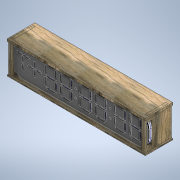
# Autodesk Inventor part: 7 Segment Clock Master
Saved by Autodesk Inventor 2021 (Build 250183000, 183)
## iProperties
Created: 2020-06-26
Part Number: 7 Segment Clock Master
Material: PMMA PlasticBlack
Document SubType Name: Modeling
Designer: dech3
Density: 1.188 g/cm^3
Appearance: Polycarbonate - Clear(1)
Author: dech3
Autodesk Inventor part; units mm, degrees
(part 1 of 5)
ref_plane "YZ Plane" through (0, 0, 0) normal (1, 0, 0) x (0, 1, 0)
ref_plane "XZ Plane" through (0, 0, 0) normal (0, 1, 0) x (-1, 0, 0)
ref_plane "XY Plane" through (0, 0, 0) normal (0, 0, 1) x (1, 0, 0)
sketch "Single Segment" plane through (0, 0, 0) normal (0, 0, 1) x (1, 0, 0)
  arc A0 (128.9839, -2.0293) -> (129.691, -2.3222) centre (129.691, -1.3222) ccw
  arc A1 (129.691, 2.6778) -> (128.9839, 2.3849) centre (129.691, 1.6778) ccw
  line L0 (128.9839, -2.0293) -> (127.0768, -0.1222)
  line L1 (128.9839, 2.3849) -> (127.0768, 0.4778)
  line L2 (127.0768, 0.1778) -> (127.0768, -0.1222)
  line L3 (127.0768, 0.1778) -> (127.0768, 0.4778)
  line L4 (129.691, 2.6778) -> (146.4626, 2.6778)
  line L5 (146.4626, -2.3222) -> (129.691, -2.3222)
  arc A2 (147.1697, 2.3849) -> (146.4626, 2.6778) centre (146.4626, 1.6778) ccw
  line L6 (147.1697, 2.3849) -> (149.0768, 0.4778)
  line L7 (149.0768, 0.1778) -> (149.0768, 0.4778)
  line L8 (149.0768, 0.1778) -> (149.0768, -0.1222)
  arc A3 (146.4626, -2.3222) -> (147.1697, -2.0293) centre (146.4626, -1.3222) ccw
  line L9 (147.1697, -2.0293) -> (149.0768, -0.1222)
  point P0 (153.0768, 0)
  point P1 (129.2768, -2.3222)
  point P2 (129.2768, 2.6778)
  point P3 (146.8768, 2.6778)
  point P4 (146.8768, -2.3222)
  dimension "d105" = 2.2
  dimension "d108" = 2.2
  dimension "d111" = 2.2
  dimension "d112" = 2.2
  dimension "d113" = 2.2
  dimension "d114" = 2.2
  dimension "d115" = 2.2
  dimension "d116" = 1
  dimension "d117" = 5
  dimension "d121" = 2.2
  dimension "d122" = 2.2
  dimension "d126" = 135
  dimension "d127" = 22
  dimension "d128" = 135
  dimension "d129" = 2.5
  dimension "d348" = 5
  dimension "d349" = 22
  dimension "d350" = 2.2
  dimension "d352" = 0.3
  dimension "d353" = 0.3
  dimension "d358" = 0.3
  dimension "d359" = 0.3
  measures "d105" horizontal distance of point (129.277, -2.322) L0.end
  measures "d108" horizontal distance of L7.end point (146.877, 2.678)
  measures "d111" horizontal distance of point (129.277, 2.678) L3.end
  measures "d112" horizontal distance of L9.end point (146.877, -2.322)
  measures "d113" horizontal distance of L9.end point (146.877, -2.322)
  measures "d114" horizontal distance of point (129.277, 2.678) L3.end
  measures "d115" horizontal distance of point (129.277, -2.322) L0.end
  measures "d116" radius of A1
  measures "d117" distance of point (146.877, -2.322) point (146.877, 2.678)
  measures "d121" horizontal distance of L7.end point (146.877, 2.678)
  measures "d122" horizontal distance of point (146.877, -2.322) L8.start
  measures "d126" angle of L5 L9
  measures "d127" horizontal distance of L9.end L3.start
  measures "d128" angle of L4 L6
  measures "d129" vertical distance of L8.start point (146.877, -2.322)
  measures "d348" distance between parallel lines of L5 L4
  measures "d349" distance of L3.start L8.start
  measures "d350" horizontal distance of point (129.277, 2.678) L3.start
  measures "d352" distance of L8.start L7.end
  measures "d353" distance of L9.end L8.start
  measures "d358" distance of L3.end L3.start
  measures "d359" distance of L0.end L3.start
sketch "7 Segment Digit" plane through (0, 0, 0) normal (0, 0, 1) x (1, 0, 0)
  arc A0 (215.9071, -11.0293) -> (216.6142, -11.3222) centre (216.6142, -10.3222) ccw
  arc A1 (216.6142, -6.3222) -> (215.9071, -6.6151) centre (216.6142, -7.3222) ccw
  line L0 (215.9071, -11.0293) -> (214, -9.1222)
  line L1 (215.9071, -6.6151) -> (214, -8.5222)
  line L2 (214, -8.8222) -> (214, -9.1222)
  line L3 (214, -8.8222) -> (214, -8.5222)
  line L4 (216.6142, -6.3222) -> (233.3858, -6.3222)
  line L5 (233.3858, -11.3222) -> (216.6142, -11.3222)
  arc A2 (234.0929, -6.6151) -> (233.3858, -6.3222) centre (233.3858, -7.3222) ccw
  line L6 (234.0929, -6.6151) -> (236, -8.5222)
  line L7 (236, -8.8222) -> (236, -8.5222)
  line L8 (236, -8.8222) -> (236, -9.1222)
  arc A3 (233.3858, -11.3222) -> (234.0929, -11.0293) centre (233.3858, -10.3222) ccw
  line L9 (234.0929, -11.0293) -> (236, -9.1222)
  arc A4 (215.9071, -35.8293) -> (216.6142, -36.1222) centre (216.6142, -35.1222) ccw
  arc A5 (216.6142, -31.1222) -> (215.9071, -31.4151) centre (216.6142, -32.1222) ccw
  line L10 (215.9071, -35.8293) -> (214, -33.9222)
  line L11 (215.9071, -31.4151) -> (214, -33.3222)
  line L12 (214, -33.6222) -> (214, -33.9222)
  line L13 (214, -33.6222) -> (214, -33.3222)
  line L14 (216.6142, -31.1222) -> (233.3858, -31.1222)
  line L15 (233.3858, -36.1222) -> (216.6142, -36.1222)
  arc A6 (234.0929, -31.4151) -> (233.3858, -31.1222) centre (233.3858, -32.1222) ccw
  line L16 (234.0929, -31.4151) -> (236, -33.3222)
  line L17 (236, -33.6222) -> (236, -33.3222)
  line L18 (236, -33.6222) -> (236, -33.9222)
  arc A7 (233.3858, -36.1222) -> (234.0929, -35.8293) centre (233.3858, -35.1222) ccw
  line L19 (234.0929, -35.8293) -> (236, -33.9222)
  arc A8 (214.8071, -30.3151) -> (215.1, -29.608) centre (214.1, -29.608) ccw
  arc A9 (210.1, -29.608) -> (210.3929, -30.3151) centre (211.1, -29.608) ccw
  line L20 (214.8071, -30.3151) -> (212.9, -32.2222)
  line L21 (210.3929, -30.3151) -> (212.3, -32.2222)
  line L22 (212.6, -32.2222) -> (212.9, -32.2222)
  line L23 (212.6, -32.2222) -> (212.3, -32.2222)
  line L24 (210.1, -29.608) -> (210.1, -12.8364)
  line L25 (215.1, -12.8364) -> (215.1, -29.608)
  arc A10 (210.3929, -12.1293) -> (210.1, -12.8364) centre (211.1, -12.8364) ccw
  line L26 (210.3929, -12.1293) -> (212.3, -10.2222)
  line L27 (212.6, -10.2222) -> (212.3, -10.2222)
  line L28 (212.6, -10.2222) -> (212.9, -10.2222)
  arc A11 (215.1, -12.8364) -> (214.8071, -12.1293) centre (214.1, -12.8364) ccw
  line L29 (214.8071, -12.1293) -> (212.9, -10.2222)
  arc A12 (214.8071, -55.1151) -> (215.1, -54.408) centre (214.1, -54.408) ccw
  arc A13 (210.1, -54.408) -> (210.3929, -55.1151) centre (211.1, -54.408) ccw
  line L30 (214.8071, -55.1151) -> (212.9, -57.0222)
  line L31 (210.3929, -55.1151) -> (212.3, -57.0222)
  line L32 (212.6, -57.0222) -> (212.9, -57.0222)
  line L33 (212.6, -57.0222) -> (212.3, -57.0222)
  line L34 (210.1, -54.408) -> (210.1, -37.6364)
  line L35 (215.1, -37.6364) -> (215.1, -54.408)
  arc A14 (210.3929, -36.9293) -> (210.1, -37.6364) centre (211.1, -37.6364) ccw
  line L36 (210.3929, -36.9293) -> (212.3, -35.0222)
  line L37 (212.6, -35.0222) -> (212.3, -35.0222)
  line L38 (212.6, -35.0222) -> (212.9, -35.0222)
  arc A15 (215.1, -37.6364) -> (214.8071, -36.9293) centre (214.1, -37.6364) ccw
  line L39 (214.8071, -36.9293) -> (212.9, -35.0222)
  arc A16 (239.6071, -30.3151) -> (239.9, -29.608) centre (238.9, -29.608) ccw
  arc A17 (234.9, -29.608) -> (235.1929, -30.3151) centre (235.9, -29.608) ccw
  line L40 (239.6071, -30.3151) -> (237.7, -32.2222)
  line L41 (235.1929, -30.3151) -> (237.1, -32.2222)
  line L42 (237.4, -32.2222) -> (237.7, -32.2222)
  line L43 (237.4, -32.2222) -> (237.1, -32.2222)
  line L44 (234.9, -29.608) -> (234.9, -12.8364)
  line L45 (239.9, -12.8364) -> (239.9, -29.608)
  arc A18 (235.1929, -12.1293) -> (234.9, -12.8364) centre (235.9, -12.8364) ccw
  line L46 (235.1929, -12.1293) -> (237.1, -10.2222)
  line L47 (237.4, -10.2222) -> (237.1, -10.2222)
  line L48 (237.4, -10.2222) -> (237.7, -10.2222)
  arc A19 (239.9, -12.8364) -> (239.6071, -12.1293) centre (238.9, -12.8364) ccw
  line L49 (239.6071, -12.1293) -> (237.7, -10.2222)
  arc A20 (239.6071, -55.1151) -> (239.9, -54.408) centre (238.9, -54.408) ccw
  arc A21 (234.9, -54.408) -> (235.1929, -55.1151) centre (235.9, -54.408) ccw
  line L50 (239.6071, -55.1151) -> (237.7, -57.0222)
  line L51 (235.1929, -55.1151) -> (237.1, -57.0222)
  line L52 (237.4, -57.0222) -> (237.7, -57.0222)
  line L53 (237.4, -57.0222) -> (237.1, -57.0222)
  line L54 (234.9, -54.408) -> (234.9, -37.6364)
  line L55 (239.9, -37.6364) -> (239.9, -54.408)
  arc A22 (235.1929, -36.9293) -> (234.9, -37.6364) centre (235.9, -37.6364) ccw
  line L56 (235.1929, -36.9293) -> (237.1, -35.0222)
  line L57 (237.4, -35.0222) -> (237.1, -35.0222)
  line L58 (237.4, -35.0222) -> (237.7, -35.0222)
  arc A23 (239.9, -37.6364) -> (239.6071, -36.9293) centre (238.9, -37.6364) ccw
  line L59 (239.6071, -36.9293) -> (237.7, -35.0222)
  arc A24 (215.9071, -60.6293) -> (216.6142, -60.9222) centre (216.6142, -59.9222) ccw
  arc A25 (216.6142, -55.9222) -> (215.9071, -56.2151) centre (216.6142, -56.9222) ccw
  line L60 (215.9071, -60.6293) -> (214, -58.7222)
  line L61 (215.9071, -56.2151) -> (214, -58.1222)
  line L62 (214, -58.4222) -> (214, -58.7222)
  line L63 (214, -58.4222) -> (214, -58.1222)
  line L64 (216.6142, -55.9222) -> (233.3858, -55.9222)
  line L65 (233.3858, -60.9222) -> (216.6142, -60.9222)
  arc A26 (234.0929, -56.2151) -> (233.3858, -55.9222) centre (233.3858, -56.9222) ccw
  line L66 (234.0929, -56.2151) -> (236, -58.1222)
  line L67 (236, -58.4222) -> (236, -58.1222)
  line L68 (236, -58.4222) -> (236, -58.7222)
  arc A27 (233.3858, -60.9222) -> (234.0929, -60.6293) centre (233.3858, -59.9222) ccw
  line L69 (234.0929, -60.6293) -> (236, -58.7222)
  point P0 (239.8857, -4.9143)
  dimension "d131" = 1.1
  dimension "d132" = 1.1
  dimension "d137" = 1.1
  dimension "d138" = 1.1
  dimension "d139" = 1.1
  dimension "d140" = 1.1
  dimension "d141" = 1.1
  dimension "d142" = 1.1
  dimension "d143" = 1.1
  dimension "d144" = 1.1
  dimension "d145" = 1.1
  dimension "d146" = 1.1
  dimension "d150" = 1.1
  dimension "d151" = 1.1
  dimension "d152" = 1.1
  dimension "d153" = 1.1
sketch "Slanted Segment Large" plane through (0, 0, 0) normal (0, 0, 1) x (1, 0, 0)
  line L0 (-252.8296, -124.6537) -> (-254.4296, -124.6537)
  line L1 (-254.4296, -124.6537) -> (-257.6296, -127.8537)
  line L2 (-257.6296, -127.8537) -> (-261.6917, -184.8537)
  line L3 (-253.6917, -184.8537) -> (-249.6296, -127.8537)
  line L4 (-249.6296, -127.8537) -> (-252.8296, -124.6537)
  line L5 (-261.6917, -184.8537) -> (-258.4917, -188.0537)
  line L6 (-258.4917, -188.0537) -> (-256.8917, -188.0537)
  line L7 (-256.8917, -188.0537) -> (-253.6917, -184.8537)
  point P0 (-253.3255, -154.094)
  point P1 (-253.6296, -124.6537)
  dimension "d294" = 3.2
  dimension "d295" = 3.2
  dimension "d296" = 8
  dimension "d297" = 3.2
  dimension "d298" = 3.2
  dimension "d299" = 57
  dimension "d304" = 3.2
  dimension "d305" = 3.2
  dimension "d306" = 3.2
  dimension "d307" = 3.2
  measures "d294" horizontal distance of L0.end L1.end
  measures "d295" horizontal distance of L3.end L0.start
  measures "d296" distance of L3.end L1.end
  measures "d297" horizontal distance of L3.end L0.start
  measures "d298" horizontal distance of L0.end L1.end
  measures "d299" vertical distance of L3.end L3.start
  measures "d304" horizontal distance of L5.end L2.end
  measures "d305" horizontal distance of L3.start L6.end
  measures "d306" horizontal distance of L2.end L5.end
  measures "d307" horizontal distance of L3.start L6.end
sketch "+ sign" plane through (0, 0, 0) normal (0, 0, 1) x (1, 0, 0)
  arc A0 (1.761, -2.8041) -> (2.4681, -3.097) centre (2.4681, -2.097) ccw
  arc A1 (2.4681, 1.903) -> (1.761, 1.6102) centre (2.4681, 0.903) ccw
  line L0 (1.761, -2.8041) -> (-0.1461, -0.897)
  line L1 (-0.1461, -0.597) -> (-0.1461, -0.297)
  line L2 (-0.1461, -0.597) -> (-0.1461, -0.897)
  line L3 (1.761, 1.6102) -> (-0.1461, -0.297)
  line L4 (2.4681, 1.903) -> (13.2397, 1.903)
  line L5 (13.2397, -3.097) -> (2.4681, -3.097)
  arc A2 (13.9468, 1.6102) -> (13.2397, 1.903) centre (13.2397, 0.903) ccw
  arc A3 (13.2397, -3.097) -> (13.9468, -2.8041) centre (13.2397, -2.097) ccw
  line L6 (13.9468, -2.8041) -> (15.8539, -0.897)
  line L7 (15.8539, -0.597) -> (15.8539, -0.897)
  line L8 (15.8539, -0.597) -> (15.8539, -0.297)
  line L9 (13.9468, 1.6102) -> (15.8539, -0.297)
  arc A4 (1.061, 2.3102) -> (1.3539, 3.0173) centre (0.3539, 3.0173) ccw
  arc A5 (-3.6461, 3.0173) -> (-3.3532, 2.3102) centre (-2.6461, 3.0173) ccw
  line L10 (1.061, 2.3102) -> (-0.8461, 0.403)
  line L11 (-1.1461, 0.403) -> (-1.4461, 0.403)
  line L12 (-1.1461, 0.403) -> (-0.8461, 0.403)
  line L13 (-3.3532, 2.3102) -> (-1.4461, 0.403)
  line L14 (-3.6461, 3.0173) -> (-3.6461, 13.7888)
  line L15 (1.3539, 13.7888) -> (1.3539, 3.0173)
  arc A6 (-3.3532, 14.4959) -> (-3.6461, 13.7888) centre (-2.6461, 13.7888) ccw
  arc A7 (1.3539, 13.7888) -> (1.061, 14.4959) centre (0.3539, 13.7888) ccw
  line L16 (1.061, 14.4959) -> (-0.8461, 16.403)
  line L17 (-1.1461, 16.403) -> (-0.8461, 16.403)
  line L18 (-1.1461, 16.403) -> (-1.4461, 16.403)
  line L19 (-3.3532, 14.4959) -> (-1.4461, 16.403)
  arc A8 (-16.239, -2.8041) -> (-15.5319, -3.097) centre (-15.5319, -2.097) ccw
  arc A9 (-15.5319, 1.903) -> (-16.239, 1.6102) centre (-15.5319, 0.903) ccw
  line L20 (-16.239, -2.8041) -> (-18.1461, -0.897)
  line L21 (-18.1461, -0.597) -> (-18.1461, -0.297)
  line L22 (-18.1461, -0.597) -> (-18.1461, -0.897)
  line L23 (-16.239, 1.6102) -> (-18.1461, -0.297)
  line L24 (-15.5319, 1.903) -> (-4.7603, 1.903)
  line L25 (-4.7603, -3.097) -> (-15.5319, -3.097)
  arc A10 (-4.0532, 1.6102) -> (-4.7603, 1.903) centre (-4.7603, 0.903) ccw
  arc A11 (-4.7603, -3.097) -> (-4.0532, -2.8041) centre (-4.7603, -2.097) ccw
  line L26 (-4.0532, -2.8041) -> (-2.1461, -0.897)
  line L27 (-2.1461, -0.597) -> (-2.1461, -0.897)
  line L28 (-2.1461, -0.597) -> (-2.1461, -0.297)
  line L29 (-4.0532, 1.6102) -> (-2.1461, -0.297)
  arc A12 (1.061, -15.6898) -> (1.3539, -14.9827) centre (0.3539, -14.9827) ccw
  arc A13 (-3.6461, -14.9827) -> (-3.3532, -15.6898) centre (-2.6461, -14.9827) ccw
  line L30 (1.061, -15.6898) -> (-0.8461, -17.597)
  line L31 (-1.1461, -17.597) -> (-1.4461, -17.597)
  line L32 (-1.1461, -17.597) -> (-0.8461, -17.597)
  line L33 (-3.3532, -15.6898) -> (-1.4461, -17.597)
  line L34 (-3.6461, -14.9827) -> (-3.6461, -4.2112)
  line L35 (1.3539, -4.2112) -> (1.3539, -14.9827)
  arc A14 (-3.3532, -3.5041) -> (-3.6461, -4.2112) centre (-2.6461, -4.2112) ccw
  arc A15 (1.3539, -4.2112) -> (1.061, -3.5041) centre (0.3539, -4.2112) ccw
  line L36 (1.061, -3.5041) -> (-0.8461, -1.597)
  line L37 (-1.1461, -1.597) -> (-0.8461, -1.597)
  line L38 (-1.1461, -1.597) -> (-1.4461, -1.597)
  line L39 (-3.3532, -3.5041) -> (-1.4461, -1.597)
  point P0 (-225.4266, -6.7349)
  dimension "d496" = 2
  dimension "d497" = 2
  dimension "d501" = 1
  dimension "d502" = 1
  dimension "d503" = 0
  dimension "d504" = 0
  dimension "d505" = 0.99
  dimension "d506" = 0.99
  dimension "d507" = 0.99
  dimension "d508" = 0.99
sketch "Dot" plane through (0, 0, 0) normal (0, 0, 1) x (1, 0, 0)
  line L0 (-36.1663, 28.3091) -> (-35.1663, 28.3091)
  line L1 (-35.1663, 28.3091) -> (-33.1663, 26.3091)
  line L2 (-33.1663, 26.3091) -> (-33.1663, 25.3091)
  line L3 (-33.1663, 25.3091) -> (-35.1663, 23.3091)
  line L4 (-35.1663, 23.3091) -> (-36.1663, 23.3091)
  line L5 (-36.1663, 23.3091) -> (-38.1663, 25.3091)
  line L6 (-38.1663, 25.3091) -> (-38.1663, 26.3091)
  line L7 (-38.1663, 26.3091) -> (-36.1663, 28.3091)
  point P0 (-33.9663, 25.3091)
  dimension "d311" = 2
  dimension "d312" = 2
  dimension "d314" = 2
  dimension "d315" = 2
  dimension "d316" = 2
  dimension "d317" = 2
  dimension "d318" = 2
  dimension "d319" = 2
  dimension "d320" = 1
  dimension "d321" = 1
  dimension "d322" = 1
  dimension "d323" = 1
  dimension "d360" = 5
  dimension "d361" = 5
  measures "d311" horizontal distance of L1.end L0.end
  measures "d312" horizontal distance of L0.start L6.end
  measures "d314" horizontal distance of L0.start L6.end
  measures "d315" horizontal distance of L1.end L0.end
  measures "d316" horizontal distance of L4.end L5.end
  measures "d317" horizontal distance of L2.end L3.end
  measures "d318" horizontal distance of L2.end L3.end
  measures "d319" horizontal distance of L5.end L4.end
  measures "d320" distance of L1.end L2.end
  measures "d321" distance of L0.end L0.start
  measures "d322" distance of L3.end L4.end
  measures "d323" distance of L6.end L5.end
  measures "d360" distance between parallel lines of L4 L0
  measures "d361" distance between parallel lines of L2 L6
sketch "Clock Face with T +-" plane through (0, 0, 0) normal (0, 0, 1) x (1, 0, 0)
  arc A0 (62.5844, 18.2447) -> (63.2916, 17.9519) centre (63.2916, 18.9519) ccw
  arc A1 (63.2916, 22.9519) -> (62.5844, 22.659) centre (63.2916, 21.9519) ccw
  line L0 (62.5844, 18.2447) -> (60.6773, 20.1519)
  line L1 (62.5844, 22.659) -> (60.6773, 20.7519)
  line L2 (60.6773, 20.4519) -> (60.6773, 20.1519)
  line L3 (60.6773, 20.4519) -> (60.6773, 20.7519)
  line L4 (63.2916, 22.9519) -> (80.0631, 22.9519)
  line L5 (80.0631, 17.9519) -> (63.2916, 17.9519)
  arc A2 (80.7702, 22.659) -> (80.0631, 22.9519) centre (80.0631, 21.9519) ccw
  line L6 (80.7702, 22.659) -> (82.6773, 20.7519)
  line L7 (82.6773, 20.4519) -> (82.6773, 20.7519)
  line L8 (82.6773, 20.4519) -> (82.6773, 20.1519)
  arc A3 (80.0631, 17.9519) -> (80.7702, 18.2447) centre (80.0631, 18.9519) ccw
  line L9 (80.7702, 18.2447) -> (82.6773, 20.1519)
  arc A4 (62.5844, -6.5553) -> (63.2916, -6.8481) centre (63.2916, -5.8481) ccw
  arc A5 (63.2916, -1.8481) -> (62.5844, -2.141) centre (63.2916, -2.8481) ccw
  line L10 (62.5844, -6.5553) -> (60.6773, -4.6481)
  line L11 (62.5844, -2.141) -> (60.6773, -4.0481)
  line L12 (60.6773, -4.3481) -> (60.6773, -4.6481)
  line L13 (60.6773, -4.3481) -> (60.6773, -4.0481)
  line L14 (63.2916, -1.8481) -> (80.0631, -1.8481)
  line L15 (80.0631, -6.8481) -> (63.2916, -6.8481)
  arc A6 (80.7702, -2.141) -> (80.0631, -1.8481) centre (80.0631, -2.8481) ccw
  line L16 (80.7702, -2.141) -> (82.6773, -4.0481)
  line L17 (82.6773, -4.3481) -> (82.6773, -4.0481)
  line L18 (82.6773, -4.3481) -> (82.6773, -4.6481)
  arc A7 (80.0631, -6.8481) -> (80.7702, -6.5553) centre (80.0631, -5.8481) ccw
  line L19 (80.7702, -6.5553) -> (82.6773, -4.6481)
  arc A8 (61.4844, -1.041) -> (61.7773, -0.3339) centre (60.7773, -0.3339) ccw
  arc A9 (56.7773, -0.3339) -> (57.0702, -1.041) centre (57.7773, -0.3339) ccw
  line L20 (61.4844, -1.041) -> (59.5773, -2.9481)
  line L21 (57.0702, -1.041) -> (58.9773, -2.9481)
  line L22 (59.2773, -2.9481) -> (59.5773, -2.9481)
  line L23 (59.2773, -2.9481) -> (58.9773, -2.9481)
  line L24 (56.7773, -0.3339) -> (56.7773, 16.4376)
  line L25 (61.7773, 16.4376) -> (61.7773, -0.3339)
  arc A10 (57.0702, 17.1447) -> (56.7773, 16.4376) centre (57.7773, 16.4376) ccw
  line L26 (57.0702, 17.1447) -> (58.9773, 19.0519)
  line L27 (59.2773, 19.0519) -> (58.9773, 19.0519)
  line L28 (59.2773, 19.0519) -> (59.5773, 19.0519)
  arc A11 (61.7773, 16.4376) -> (61.4844, 17.1447) centre (60.7773, 16.4376) ccw
  line L29 (61.4844, 17.1447) -> (59.5773, 19.0519)
  arc A12 (61.4844, -25.841) -> (61.7773, -25.1339) centre (60.7773, -25.1339) ccw
  arc A13 (56.7773, -25.1339) -> (57.0702, -25.841) centre (57.7773, -25.1339) ccw
  line L30 (61.4844, -25.841) -> (59.5773, -27.7481)
  line L31 (57.0702, -25.841) -> (58.9773, -27.7481)
  line L32 (59.2773, -27.7481) -> (59.5773, -27.7481)
  line L33 (59.2773, -27.7481) -> (58.9773, -27.7481)
  line L34 (56.7773, -25.1339) -> (56.7773, -8.3624)
  line L35 (61.7773, -8.3624) -> (61.7773, -25.1339)
  arc A14 (57.0702, -7.6553) -> (56.7773, -8.3624) centre (57.7773, -8.3624) ccw
  line L36 (57.0702, -7.6553) -> (58.9773, -5.7481)
  line L37 (59.2773, -5.7481) -> (58.9773, -5.7481)
  line L38 (59.2773, -5.7481) -> (59.5773, -5.7481)
  arc A15 (61.7773, -8.3624) -> (61.4844, -7.6553) centre (60.7773, -8.3624) ccw
  line L39 (61.4844, -7.6553) -> (59.5773, -5.7481)
  arc A16 (86.2844, -1.041) -> (86.5773, -0.3339) centre (85.5773, -0.3339) ccw
  arc A17 (81.5773, -0.3339) -> (81.8702, -1.041) centre (82.5773, -0.3339) ccw
  line L40 (86.2844, -1.041) -> (84.3773, -2.9481)
  line L41 (81.8702, -1.041) -> (83.7773, -2.9481)
  line L42 (84.0773, -2.9481) -> (84.3773, -2.9481)
  line L43 (84.0773, -2.9481) -> (83.7773, -2.9481)
  line L44 (81.5773, -0.3339) -> (81.5773, 16.4376)
  line L45 (86.5773, 16.4376) -> (86.5773, -0.3339)
  arc A18 (81.8702, 17.1447) -> (81.5773, 16.4376) centre (82.5773, 16.4376) ccw
  line L46 (81.8702, 17.1447) -> (83.7773, 19.0519)
  line L47 (84.0773, 19.0519) -> (83.7773, 19.0519)
  line L48 (84.0773, 19.0519) -> (84.3773, 19.0519)
  arc A19 (86.5773, 16.4376) -> (86.2844, 17.1447) centre (85.5773, 16.4376) ccw
  line L49 (86.2844, 17.1447) -> (84.3773, 19.0519)
  arc A20 (86.2844, -25.841) -> (86.5773, -25.1339) centre (85.5773, -25.1339) ccw
  arc A21 (81.5773, -25.1339) -> (81.8702, -25.841) centre (82.5773, -25.1339) ccw
  line L50 (86.2844, -25.841) -> (84.3773, -27.7481)
  line L51 (81.8702, -25.841) -> (83.7773, -27.7481)
  line L52 (84.0773, -27.7481) -> (84.3773, -27.7481)
  line L53 (84.0773, -27.7481) -> (83.7773, -27.7481)
  line L54 (81.5773, -25.1339) -> (81.5773, -8.3624)
  line L55 (86.5773, -8.3624) -> (86.5773, -25.1339)
  arc A22 (81.8702, -7.6553) -> (81.5773, -8.3624) centre (82.5773, -8.3624) ccw
  line L56 (81.8702, -7.6553) -> (83.7773, -5.7481)
  line L57 (84.0773, -5.7481) -> (83.7773, -5.7481)
  line L58 (84.0773, -5.7481) -> (84.3773, -5.7481)
  arc A23 (86.5773, -8.3624) -> (86.2844, -7.6553) centre (85.5773, -8.3624) ccw
  line L59 (86.2844, -7.6553) -> (84.3773, -5.7481)
  arc A24 (62.5844, -31.3553) -> (63.2916, -31.6481) centre (63.2916, -30.6481) ccw
  arc A25 (63.2916, -26.6481) -> (62.5844, -26.941) centre (63.2916, -27.6481) ccw
  line L60 (62.5844, -31.3553) -> (60.6773, -29.4481)
  line L61 (62.5844, -26.941) -> (60.6773, -28.8481)
  line L62 (60.6773, -29.1481) -> (60.6773, -29.4481)
  line L63 (60.6773, -29.1481) -> (60.6773, -28.8481)
  line L64 (63.2916, -26.6481) -> (80.0631, -26.6481)
  line L65 (80.0631, -31.6481) -> (63.2916, -31.6481)
  arc A26 (80.7702, -26.941) -> (80.0631, -26.6481) centre (80.0631, -27.6481) ccw
  line L66 (80.7702, -26.941) -> (82.6773, -28.8481)
  line L67 (82.6773, -29.1481) -> (82.6773, -28.8481)
  line L68 (82.6773, -29.1481) -> (82.6773, -29.4481)
  arc A27 (80.0631, -31.6481) -> (80.7702, -31.3553) centre (80.0631, -30.6481) ccw
  line L69 (80.7702, -31.3553) -> (82.6773, -29.4481)
  arc A28 (15.7844, 18.2447) -> (16.4916, 17.9519) centre (16.4916, 18.9519) ccw
  arc A29 (16.4916, 22.9519) -> (15.7844, 22.659) centre (16.4916, 21.9519) ccw
  line L70 (15.7844, 18.2447) -> (13.8773, 20.1519)
  line L71 (15.7844, 22.659) -> (13.8773, 20.7519)
  line L72 (13.8773, 20.4519) -> (13.8773, 20.1519)
  line L73 (13.8773, 20.4519) -> (13.8773, 20.7519)
  line L74 (16.4916, 22.9519) -> (33.2631, 22.9519)
  line L75 (33.2631, 17.9519) -> (16.4916, 17.9519)
  arc A30 (33.9702, 22.659) -> (33.2631, 22.9519) centre (33.2631, 21.9519) ccw
  line L76 (33.9702, 22.659) -> (35.8773, 20.7519)
  line L77 (35.8773, 20.4519) -> (35.8773, 20.7519)
  line L78 (35.8773, 20.4519) -> (35.8773, 20.1519)
  arc A31 (33.2631, 17.9519) -> (33.9702, 18.2447) centre (33.2631, 18.9519) ccw
  line L79 (33.9702, 18.2447) -> (35.8773, 20.1519)
  arc A32 (15.7844, -6.5553) -> (16.4916, -6.8481) centre (16.4916, -5.8481) ccw
  arc A33 (16.4916, -1.8481) -> (15.7844, -2.141) centre (16.4916, -2.8481) ccw
  line L80 (15.7844, -6.5553) -> (13.8773, -4.6481)
  line L81 (15.7844, -2.141) -> (13.8773, -4.0481)
  line L82 (13.8773, -4.3481) -> (13.8773, -4.6481)
  line L83 (13.8773, -4.3481) -> (13.8773, -4.0481)
  line L84 (16.4916, -1.8481) -> (33.2631, -1.8481)
  line L85 (33.2631, -6.8481) -> (16.4916, -6.8481)
  arc A34 (33.9702, -2.141) -> (33.2631, -1.8481) centre (33.2631, -2.8481) ccw
  line L86 (33.9702, -2.141) -> (35.8773, -4.0481)
  line L87 (35.8773, -4.3481) -> (35.8773, -4.0481)
  line L88 (35.8773, -4.3481) -> (35.8773, -4.6481)
  arc A35 (33.2631, -6.8481) -> (33.9702, -6.5553) centre (33.2631, -5.8481) ccw
  line L89 (33.9702, -6.5553) -> (35.8773, -4.6481)
  arc A36 (14.6844, -1.041) -> (14.9773, -0.3339) centre (13.9773, -0.3339) ccw
  arc A37 (9.9773, -0.3339) -> (10.2702, -1.041) centre (10.9773, -0.3339) ccw
  line L90 (14.6844, -1.041) -> (12.7773, -2.9481)
  line L91 (10.2702, -1.041) -> (12.1773, -2.9481)
  line L92 (12.4773, -2.9481) -> (12.7773, -2.9481)
  line L93 (12.4773, -2.9481) -> (12.1773, -2.9481)
  line L94 (9.9773, -0.3339) -> (9.9773, 16.4376)
  line L95 (14.9773, 16.4376) -> (14.9773, -0.3339)
  arc A38 (10.2702, 17.1447) -> (9.9773, 16.4376) centre (10.9773, 16.4376) ccw
  line L96 (10.2702, 17.1447) -> (12.1773, 19.0519)
  line L97 (12.4773, 19.0519) -> (12.1773, 19.0519)
  line L98 (12.4773, 19.0519) -> (12.7773, 19.0519)
  arc A39 (14.9773, 16.4376) -> (14.6844, 17.1447) centre (13.9773, 16.4376) ccw
  line L99 (14.6844, 17.1447) -> (12.7773, 19.0519)
  arc A40 (14.6844, -25.841) -> (14.9773, -25.1339) centre (13.9773, -25.1339) ccw
  arc A41 (9.9773, -25.1339) -> (10.2702, -25.841) centre (10.9773, -25.1339) ccw
  line L100 (14.6844, -25.841) -> (12.7773, -27.7481)
  line L101 (10.2702, -25.841) -> (12.1773, -27.7481)
  line L102 (12.4773, -27.7481) -> (12.7773, -27.7481)
  line L103 (12.4773, -27.7481) -> (12.1773, -27.7481)
  line L104 (9.9773, -25.1339) -> (9.9773, -8.3624)
  line L105 (14.9773, -8.3624) -> (14.9773, -25.1339)
  arc A42 (10.2702, -7.6553) -> (9.9773, -8.3624) centre (10.9773, -8.3624) ccw
  line L106 (10.2702, -7.6553) -> (12.1773, -5.7481)
  line L107 (12.4773, -5.7481) -> (12.1773, -5.7481)
  line L108 (12.4773, -5.7481) -> (12.7773, -5.7481)
  arc A43 (14.9773, -8.3624) -> (14.6844, -7.6553) centre (13.9773, -8.3624) ccw
  line L109 (14.6844, -7.6553) -> (12.7773, -5.7481)
  arc A44 (39.4844, -1.041) -> (39.7773, -0.3339) centre (38.7773, -0.3339) ccw
  arc A45 (34.7773, -0.3339) -> (35.0702, -1.041) centre (35.7773, -0.3339) ccw
  line L110 (39.4844, -1.041) -> (37.5773, -2.9481)
  line L111 (35.0702, -1.041) -> (36.9773, -2.9481)
  line L112 (37.2773, -2.9481) -> (37.5773, -2.9481)
  line L113 (37.2773, -2.9481) -> (36.9773, -2.9481)
  line L114 (34.7773, -0.3339) -> (34.7773, 16.4376)
  line L115 (39.7773, 16.4376) -> (39.7773, -0.3339)
  arc A46 (35.0702, 17.1447) -> (34.7773, 16.4376) centre (35.7773, 16.4376) ccw
  line L116 (35.0702, 17.1447) -> (36.9773, 19.0519)
  line L117 (37.2773, 19.0519) -> (36.9773, 19.0519)
  line L118 (37.2773, 19.0519) -> (37.5773, 19.0519)
  arc A47 (39.7773, 16.4376) -> (39.4844, 17.1447) centre (38.7773, 16.4376) ccw
  line L119 (39.4844, 17.1447) -> (37.5773, 19.0519)
  arc A48 (39.4844, -25.841) -> (39.7773, -25.1339) centre (38.7773, -25.1339) ccw
  arc A49 (34.7773, -25.1339) -> (35.0702, -25.841) centre (35.7773, -25.1339) ccw
  line L120 (39.4844, -25.841) -> (37.5773, -27.7481)
  line L121 (35.0702, -25.841) -> (36.9773, -27.7481)
  line L122 (37.2773, -27.7481) -> (37.5773, -27.7481)
  line L123 (37.2773, -27.7481) -> (36.9773, -27.7481)
  line L124 (34.7773, -25.1339) -> (34.7773, -8.3624)
  line L125 (39.7773, -8.3624) -> (39.7773, -25.1339)
  arc A50 (35.0702, -7.6553) -> (34.7773, -8.3624) centre (35.7773, -8.3624) ccw
  line L126 (35.0702, -7.6553) -> (36.9773, -5.7481)
  line L127 (37.2773, -5.7481) -> (36.9773, -5.7481)
  line L128 (37.2773, -5.7481) -> (37.5773, -5.7481)
  arc A51 (39.7773, -8.3624) -> (39.4844, -7.6553) centre (38.7773, -8.3624) ccw
  line L129 (39.4844, -7.6553) -> (37.5773, -5.7481)
  arc A52 (15.7844, -31.3553) -> (16.4916, -31.6481) centre (16.4916, -30.6481) ccw
  arc A53 (16.4916, -26.6481) -> (15.7844, -26.941) centre (16.4916, -27.6481) ccw
  line L130 (15.7844, -31.3553) -> (13.8773, -29.4481)
  line L131 (15.7844, -26.941) -> (13.8773, -28.8481)
  line L132 (13.8773, -29.1481) -> (13.8773, -29.4481)
  line L133 (13.8773, -29.1481) -> (13.8773, -28.8481)
  line L134 (16.4916, -26.6481) -> (33.2631, -26.6481)
  line L135 (33.2631, -31.6481) -> (16.4916, -31.6481)
  arc A54 (33.9702, -26.941) -> (33.2631, -26.6481) centre (33.2631, -27.6481) ccw
  line L136 (33.9702, -26.941) -> (35.8773, -28.8481)
  line L137 (35.8773, -29.1481) -> (35.8773, -28.8481)
  line L138 (35.8773, -29.1481) -> (35.8773, -29.4481)
  arc A55 (33.2631, -31.6481) -> (33.9702, -31.3553) centre (33.2631, -30.6481) ccw
  line L139 (33.9702, -31.3553) -> (35.8773, -29.4481)
  arc A56 (-21.5156, 18.2447) -> (-20.8084, 17.9519) centre (-20.8084, 18.9519) ccw
  arc A57 (-20.8084, 22.9519) -> (-21.5156, 22.659) centre (-20.8084, 21.9519) ccw
  line L140 (-21.5156, 18.2447) -> (-23.4227, 20.1519)
  line L141 (-21.5156, 22.659) -> (-23.4227, 20.7519)
  line L142 (-23.4227, 20.4519) -> (-23.4227, 20.1519)
  line L143 (-23.4227, 20.4519) -> (-23.4227, 20.7519)
  line L144 (-20.8084, 22.9519) -> (-4.0369, 22.9519)
  line L145 (-4.0369, 17.9519) -> (-20.8084, 17.9519)
  arc A58 (-3.3298, 22.659) -> (-4.0369, 22.9519) centre (-4.0369, 21.9519) ccw
  line L146 (-3.3298, 22.659) -> (-1.4227, 20.7519)
  line L147 (-1.4227, 20.4519) -> (-1.4227, 20.7519)
  line L148 (-1.4227, 20.4519) -> (-1.4227, 20.1519)
  arc A59 (-4.0369, 17.9519) -> (-3.3298, 18.2447) centre (-4.0369, 18.9519) ccw
  line L149 (-3.3298, 18.2447) -> (-1.4227, 20.1519)
  arc A60 (-21.5156, -6.5553) -> (-20.8084, -6.8481) centre (-20.8084, -5.8481) ccw
  arc A61 (-20.8084, -1.8481) -> (-21.5156, -2.141) centre (-20.8084, -2.8481) ccw
  line L150 (-21.5156, -6.5553) -> (-23.4227, -4.6481)
  line L151 (-21.5156, -2.141) -> (-23.4227, -4.0481)
  line L152 (-23.4227, -4.3481) -> (-23.4227, -4.6481)
  line L153 (-23.4227, -4.3481) -> (-23.4227, -4.0481)
  line L154 (-20.8084, -1.8481) -> (-4.0369, -1.8481)
  line L155 (-4.0369, -6.8481) -> (-20.8084, -6.8481)
  arc A62 (-3.3298, -2.141) -> (-4.0369, -1.8481) centre (-4.0369, -2.8481) ccw
  line L156 (-3.3298, -2.141) -> (-1.4227, -4.0481)
  line L157 (-1.4227, -4.3481) -> (-1.4227, -4.0481)
  line L158 (-1.4227, -4.3481) -> (-1.4227, -4.6481)
  arc A63 (-4.0369, -6.8481) -> (-3.3298, -6.5553) centre (-4.0369, -5.8481) ccw
  line L159 (-3.3298, -6.5553) -> (-1.4227, -4.6481)
  arc A64 (-22.6156, -1.041) -> (-22.3227, -0.3339) centre (-23.3227, -0.3339) ccw
  arc A65 (-27.3227, -0.3339) -> (-27.0298, -1.041) centre (-26.3227, -0.3339) ccw
  line L160 (-22.6156, -1.041) -> (-24.5227, -2.9481)
  line L161 (-27.0298, -1.041) -> (-25.1227, -2.9481)
  line L162 (-24.8227, -2.9481) -> (-24.5227, -2.9481)
  line L163 (-24.8227, -2.9481) -> (-25.1227, -2.9481)
  line L164 (-27.3227, -0.3339) -> (-27.3227, 16.4376)
  line L165 (-22.3227, 16.4376) -> (-22.3227, -0.3339)
  arc A66 (-27.0298, 17.1447) -> (-27.3227, 16.4376) centre (-26.3227, 16.4376) ccw
  line L166 (-27.0298, 17.1447) -> (-25.1227, 19.0519)
  line L167 (-24.8227, 19.0519) -> (-25.1227, 19.0519)
  line L168 (-24.8227, 19.0519) -> (-24.5227, 19.0519)
  arc A67 (-22.3227, 16.4376) -> (-22.6156, 17.1447) centre (-23.3227, 16.4376) ccw
  line L169 (-22.6156, 17.1447) -> (-24.5227, 19.0519)
  arc A68 (-22.6156, -25.841) -> (-22.3227, -25.1339) centre (-23.3227, -25.1339) ccw
  arc A69 (-27.3227, -25.1339) -> (-27.0298, -25.841) centre (-26.3227, -25.1339) ccw
  line L170 (-22.6156, -25.841) -> (-24.5227, -27.7481)
  line L171 (-27.0298, -25.841) -> (-25.1227, -27.7481)
  line L172 (-24.8227, -27.7481) -> (-24.5227, -27.7481)
  line L173 (-24.8227, -27.7481) -> (-25.1227, -27.7481)
  line L174 (-27.3227, -25.1339) -> (-27.3227, -8.3624)
  line L175 (-22.3227, -8.3624) -> (-22.3227, -25.1339)
  arc A70 (-27.0298, -7.6553) -> (-27.3227, -8.3624) centre (-26.3227, -8.3624) ccw
  line L176 (-27.0298, -7.6553) -> (-25.1227, -5.7481)
  line L177 (-24.8227, -5.7481) -> (-25.1227, -5.7481)
  line L178 (-24.8227, -5.7481) -> (-24.5227, -5.7481)
  arc A71 (-22.3227, -8.3624) -> (-22.6156, -7.6553) centre (-23.3227, -8.3624) ccw
  line L179 (-22.6156, -7.6553) -> (-24.5227, -5.7481)
  arc A72 (2.1844, -1.041) -> (2.4773, -0.3339) centre (1.4773, -0.3339) ccw
  arc A73 (-2.5227, -0.3339) -> (-2.2298, -1.041) centre (-1.5227, -0.3339) ccw
  line L180 (2.1844, -1.041) -> (0.2773, -2.9481)
  line L181 (-2.2298, -1.041) -> (-0.3227, -2.9481)
  line L182 (-0.0227, -2.9481) -> (0.2773, -2.9481)
  line L183 (-0.0227, -2.9481) -> (-0.3227, -2.9481)
  line L184 (-2.5227, -0.3339) -> (-2.5227, 16.4376)
  line L185 (2.4773, 16.4376) -> (2.4773, -0.3339)
  arc A74 (-2.2298, 17.1447) -> (-2.5227, 16.4376) centre (-1.5227, 16.4376) ccw
  line L186 (-2.2298, 17.1447) -> (-0.3227, 19.0519)
  line L187 (-0.0227, 19.0519) -> (-0.3227, 19.0519)
  line L188 (-0.0227, 19.0519) -> (0.2773, 19.0519)
  arc A75 (2.4773, 16.4376) -> (2.1844, 17.1447) centre (1.4773, 16.4376) ccw
  line L189 (2.1844, 17.1447) -> (0.2773, 19.0519)
  arc A76 (2.1844, -25.841) -> (2.4773, -25.1339) centre (1.4773, -25.1339) ccw
  arc A77 (-2.5227, -25.1339) -> (-2.2298, -25.841) centre (-1.5227, -25.1339) ccw
  line L190 (2.1844, -25.841) -> (0.2773, -27.7481)
  line L191 (-2.2298, -25.841) -> (-0.3227, -27.7481)
  line L192 (-0.0227, -27.7481) -> (0.2773, -27.7481)
  line L193 (-0.0227, -27.7481) -> (-0.3227, -27.7481)
  line L194 (-2.5227, -25.1339) -> (-2.5227, -8.3624)
  line L195 (2.4773, -8.3624) -> (2.4773, -25.1339)
  arc A78 (-2.2298, -7.6553) -> (-2.5227, -8.3624) centre (-1.5227, -8.3624) ccw
  line L196 (-2.2298, -7.6553) -> (-0.3227, -5.7481)
  line L197 (-0.0227, -5.7481) -> (-0.3227, -5.7481)
  line L198 (-0.0227, -5.7481) -> (0.2773, -5.7481)
  arc A79 (2.4773, -8.3624) -> (2.1844, -7.6553) centre (1.4773, -8.3624) ccw
  line L199 (2.1844, -7.6553) -> (0.2773, -5.7481)
  arc A80 (-21.5156, -31.3553) -> (-20.8084, -31.6481) centre (-20.8084, -30.6481) ccw
  arc A81 (-20.8084, -26.6481) -> (-21.5156, -26.941) centre (-20.8084, -27.6481) ccw
  line L200 (-21.5156, -31.3553) -> (-23.4227, -29.4481)
  line L201 (-21.5156, -26.941) -> (-23.4227, -28.8481)
  line L202 (-23.4227, -29.1481) -> (-23.4227, -29.4481)
  line L203 (-23.4227, -29.1481) -> (-23.4227, -28.8481)
  line L204 (-20.8084, -26.6481) -> (-4.0369, -26.6481)
  line L205 (-4.0369, -31.6481) -> (-20.8084, -31.6481)
  arc A82 (-3.3298, -26.941) -> (-4.0369, -26.6481) centre (-4.0369, -27.6481) ccw
  line L206 (-3.3298, -26.941) -> (-1.4227, -28.8481)
  line L207 (-1.4227, -29.1481) -> (-1.4227, -28.8481)
  line L208 (-1.4227, -29.1481) -> (-1.4227, -29.4481)
  arc A83 (-4.0369, -31.6481) -> (-3.3298, -31.3553) centre (-4.0369, -30.6481) ccw
  line L209 (-3.3298, -31.3553) -> (-1.4227, -29.4481)
  arc A84 (-68.3156, 18.2447) -> (-67.6084, 17.9519) centre (-67.6084, 18.9519) ccw
  arc A85 (-67.6084, 22.9519) -> (-68.3156, 22.659) centre (-67.6084, 21.9519) ccw
  line L210 (-68.3156, 18.2447) -> (-70.2227, 20.1519)
  line L211 (-68.3156, 22.659) -> (-70.2227, 20.7519)
  line L212 (-70.2227, 20.4519) -> (-70.2227, 20.1519)
  line L213 (-70.2227, 20.4519) -> (-70.2227, 20.7519)
  line L214 (-67.6084, 22.9519) -> (-50.8369, 22.9519)
  line L215 (-50.8369, 17.9519) -> (-67.6084, 17.9519)
  arc A86 (-50.1298, 22.659) -> (-50.8369, 22.9519) centre (-50.8369, 21.9519) ccw
  line L216 (-50.1298, 22.659) -> (-48.2227, 20.7519)
  line L217 (-48.2227, 20.4519) -> (-48.2227, 20.7519)
  line L218 (-48.2227, 20.4519) -> (-48.2227, 20.1519)
  arc A87 (-50.8369, 17.9519) -> (-50.1298, 18.2447) centre (-50.8369, 18.9519) ccw
  line L219 (-50.1298, 18.2447) -> (-48.2227, 20.1519)
  arc A88 (-68.3156, -6.5553) -> (-67.6084, -6.8481) centre (-67.6084, -5.8481) ccw
  arc A89 (-67.6084, -1.8481) -> (-68.3156, -2.141) centre (-67.6084, -2.8481) ccw
  line L220 (-68.3156, -6.5553) -> (-70.2227, -4.6481)
  line L221 (-68.3156, -2.141) -> (-70.2227, -4.0481)
  line L222 (-70.2227, -4.3481) -> (-70.2227, -4.6481)
  line L223 (-70.2227, -4.3481) -> (-70.2227, -4.0481)
  line L224 (-67.6084, -1.8481) -> (-50.8369, -1.8481)
  line L225 (-50.8369, -6.8481) -> (-67.6084, -6.8481)
  arc A90 (-50.1298, -2.141) -> (-50.8369, -1.8481) centre (-50.8369, -2.8481) ccw
  line L226 (-50.1298, -2.141) -> (-48.2227, -4.0481)
  line L227 (-48.2227, -4.3481) -> (-48.2227, -4.0481)
  line L228 (-48.2227, -4.3481) -> (-48.2227, -4.6481)
  arc A91 (-50.8369, -6.8481) -> (-50.1298, -6.5553) centre (-50.8369, -5.8481) ccw
  line L229 (-50.1298, -6.5553) -> (-48.2227, -4.6481)
  arc A92 (-69.4156, -1.041) -> (-69.1227, -0.3339) centre (-70.1227, -0.3339) ccw
  arc A93 (-74.1227, -0.3339) -> (-73.8298, -1.041) centre (-73.1227, -0.3339) ccw
  line L230 (-69.4156, -1.041) -> (-71.3227, -2.9481)
  line L231 (-73.8298, -1.041) -> (-71.9227, -2.9481)
  line L232 (-71.6227, -2.9481) -> (-71.3227, -2.9481)
  line L233 (-71.6227, -2.9481) -> (-71.9227, -2.9481)
  line L234 (-74.1227, -0.3339) -> (-74.1227, 16.4376)
  line L235 (-69.1227, 16.4376) -> (-69.1227, -0.3339)
  arc A94 (-73.8298, 17.1447) -> (-74.1227, 16.4376) centre (-73.1227, 16.4376) ccw
  line L236 (-73.8298, 17.1447) -> (-71.9227, 19.0519)
  line L237 (-71.6227, 19.0519) -> (-71.9227, 19.0519)
  line L238 (-71.6227, 19.0519) -> (-71.3227, 19.0519)
  arc A95 (-69.1227, 16.4376) -> (-69.4156, 17.1447) centre (-70.1227, 16.4376) ccw
  line L239 (-69.4156, 17.1447) -> (-71.3227, 19.0519)
  arc A96 (-69.4156, -25.841) -> (-69.1227, -25.1339) centre (-70.1227, -25.1339) ccw
  arc A97 (-74.1227, -25.1339) -> (-73.8298, -25.841) centre (-73.1227, -25.1339) ccw
  line L240 (-69.4156, -25.841) -> (-71.3227, -27.7481)
  line L241 (-73.8298, -25.841) -> (-71.9227, -27.7481)
  line L242 (-71.6227, -27.7481) -> (-71.3227, -27.7481)
  line L243 (-71.6227, -27.7481) -> (-71.9227, -27.7481)
  line L244 (-74.1227, -25.1339) -> (-74.1227, -8.3624)
  line L245 (-69.1227, -8.3624) -> (-69.1227, -25.1339)
  arc A98 (-73.8298, -7.6553) -> (-74.1227, -8.3624) centre (-73.1227, -8.3624) ccw
  line L246 (-73.8298, -7.6553) -> (-71.9227, -5.7481)
  line L247 (-71.6227, -5.7481) -> (-71.9227, -5.7481)
  line L248 (-71.6227, -5.7481) -> (-71.3227, -5.7481)
  arc A99 (-69.1227, -8.3624) -> (-69.4156, -7.6553) centre (-70.1227, -8.3624) ccw
  line L249 (-69.4156, -7.6553) -> (-71.3227, -5.7481)
  arc A100 (-44.6156, -1.041) -> (-44.3227, -0.3339) centre (-45.3227, -0.3339) ccw
  arc A101 (-49.3227, -0.3339) -> (-49.0298, -1.041) centre (-48.3227, -0.3339) ccw
  line L250 (-44.6156, -1.041) -> (-46.5227, -2.9481)
  line L251 (-49.0298, -1.041) -> (-47.1227, -2.9481)
  line L252 (-46.8227, -2.9481) -> (-46.5227, -2.9481)
  line L253 (-46.8227, -2.9481) -> (-47.1227, -2.9481)
  line L254 (-49.3227, -0.3339) -> (-49.3227, 16.4376)
  line L255 (-44.3227, 16.4376) -> (-44.3227, -0.3339)
  arc A102 (-49.0298, 17.1447) -> (-49.3227, 16.4376) centre (-48.3227, 16.4376) ccw
  line L256 (-49.0298, 17.1447) -> (-47.1227, 19.0519)
  line L257 (-46.8227, 19.0519) -> (-47.1227, 19.0519)
  line L258 (-46.8227, 19.0519) -> (-46.5227, 19.0519)
  arc A103 (-44.3227, 16.4376) -> (-44.6156, 17.1447) centre (-45.3227, 16.4376) ccw
  line L259 (-44.6156, 17.1447) -> (-46.5227, 19.0519)
  arc A104 (-44.6156, -25.841) -> (-44.3227, -25.1339) centre (-45.3227, -25.1339) ccw
  arc A105 (-49.3227, -25.1339) -> (-49.0298, -25.841) centre (-48.3227, -25.1339) ccw
  line L260 (-44.6156, -25.841) -> (-46.5227, -27.7481)
  line L261 (-49.0298, -25.841) -> (-47.1227, -27.7481)
  line L262 (-46.8227, -27.7481) -> (-46.5227, -27.7481)
  line L263 (-46.8227, -27.7481) -> (-47.1227, -27.7481)
  line L264 (-49.3227, -25.1339) -> (-49.3227, -8.3624)
  line L265 (-44.3227, -8.3624) -> (-44.3227, -25.1339)
  arc A106 (-49.0298, -7.6553) -> (-49.3227, -8.3624) centre (-48.3227, -8.3624) ccw
  line L266 (-49.0298, -7.6553) -> (-47.1227, -5.7481)
  line L267 (-46.8227, -5.7481) -> (-47.1227, -5.7481)
  line L268 (-46.8227, -5.7481) -> (-46.5227, -5.7481)
  arc A107 (-44.3227, -8.3624) -> (-44.6156, -7.6553) centre (-45.3227, -8.3624) ccw
  line L269 (-44.6156, -7.6553) -> (-46.5227, -5.7481)
  arc A108 (-68.3156, -31.3553) -> (-67.6084, -31.6481) centre (-67.6084, -30.6481) ccw
  arc A109 (-67.6084, -26.6481) -> (-68.3156, -26.941) centre (-67.6084, -27.6481) ccw
  line L270 (-68.3156, -31.3553) -> (-70.2227, -29.4481)
  line L271 (-68.3156, -26.941) -> (-70.2227, -28.8481)
  line L272 (-70.2227, -29.1481) -> (-70.2227, -29.4481)
  line L273 (-70.2227, -29.1481) -> (-70.2227, -28.8481)
  line L274 (-67.6084, -26.6481) -> (-50.8369, -26.6481)
  line L275 (-50.8369, -31.6481) -> (-67.6084, -31.6481)
  arc A110 (-50.1298, -26.941) -> (-50.8369, -26.6481) centre (-50.8369, -27.6481) ccw
  line L276 (-50.1298, -26.941) -> (-48.2227, -28.8481)
  line L277 (-48.2227, -29.1481) -> (-48.2227, -28.8481)
  line L278 (-48.2227, -29.1481) -> (-48.2227, -29.4481)
  arc A111 (-50.8369, -31.6481) -> (-50.1298, -31.3553) centre (-50.8369, -30.6481) ccw
  line L279 (-50.1298, -31.3553) -> (-48.2227, -29.4481)
  arc A112 (-105.6156, 18.2447) -> (-104.9084, 17.9519) centre (-104.9084, 18.9519) ccw
  arc A113 (-104.9084, 22.9519) -> (-105.6156, 22.659) centre (-104.9084, 21.9519) ccw
  line L280 (-105.6156, 18.2447) -> (-107.5227, 20.1519)
  line L281 (-105.6156, 22.659) -> (-107.5227, 20.7519)
  line L282 (-107.5227, 20.4519) -> (-107.5227, 20.1519)
  line L283 (-107.5227, 20.4519) -> (-107.5227, 20.7519)
  line L284 (-104.9084, 22.9519) -> (-88.1369, 22.9519)
  line L285 (-88.1369, 17.9519) -> (-104.9084, 17.9519)
  arc A114 (-87.4298, 22.659) -> (-88.1369, 22.9519) centre (-88.1369, 21.9519) ccw
  line L286 (-87.4298, 22.659) -> (-85.5227, 20.7519)
  line L287 (-85.5227, 20.4519) -> (-85.5227, 20.7519)
  line L288 (-85.5227, 20.4519) -> (-85.5227, 20.1519)
  arc A115 (-88.1369, 17.9519) -> (-87.4298, 18.2447) centre (-88.1369, 18.9519) ccw
  line L289 (-87.4298, 18.2447) -> (-85.5227, 20.1519)
  arc A116 (-105.6156, -6.5553) -> (-104.9084, -6.8481) centre (-104.9084, -5.8481) ccw
  arc A117 (-104.9084, -1.8481) -> (-105.6156, -2.141) centre (-104.9084, -2.8481) ccw
  line L290 (-105.6156, -6.5553) -> (-107.5227, -4.6481)
  line L291 (-105.6156, -2.141) -> (-107.5227, -4.0481)
  line L292 (-107.5227, -4.3481) -> (-107.5227, -4.6481)
  line L293 (-107.5227, -4.3481) -> (-107.5227, -4.0481)
  line L294 (-104.9084, -1.8481) -> (-88.1369, -1.8481)
  line L295 (-88.1369, -6.8481) -> (-104.9084, -6.8481)
  arc A118 (-87.4298, -2.141) -> (-88.1369, -1.8481) centre (-88.1369, -2.8481) ccw
  line L296 (-87.4298, -2.141) -> (-85.5227, -4.0481)
  line L297 (-85.5227, -4.3481) -> (-85.5227, -4.0481)
  line L298 (-85.5227, -4.3481) -> (-85.5227, -4.6481)
  arc A119 (-88.1369, -6.8481) -> (-87.4298, -6.5553) centre (-88.1369, -5.8481) ccw
  line L299 (-87.4298, -6.5553) -> (-85.5227, -4.6481)
  arc A120 (-106.7156, -1.041) -> (-106.4227, -0.3339) centre (-107.4227, -0.3339) ccw
  arc A121 (-111.4227, -0.3339) -> (-111.1298, -1.041) centre (-110.4227, -0.3339) ccw
  line L300 (-106.7156, -1.041) -> (-108.6227, -2.9481)
  line L301 (-111.1298, -1.041) -> (-109.2227, -2.9481)
  line L302 (-108.9227, -2.9481) -> (-108.6227, -2.9481)
  line L303 (-108.9227, -2.9481) -> (-109.2227, -2.9481)
  line L304 (-111.4227, -0.3339) -> (-111.4227, 16.4376)
  line L305 (-106.4227, 16.4376) -> (-106.4227, -0.3339)
  arc A122 (-111.1298, 17.1447) -> (-111.4227, 16.4376) centre (-110.4227, 16.4376) ccw
  line L306 (-111.1298, 17.1447) -> (-109.2227, 19.0519)
  line L307 (-108.9227, 19.0519) -> (-109.2227, 19.0519)
  line L308 (-108.9227, 19.0519) -> (-108.6227, 19.0519)
  arc A123 (-106.4227, 16.4376) -> (-106.7156, 17.1447) centre (-107.4227, 16.4376) ccw
  line L309 (-106.7156, 17.1447) -> (-108.6227, 19.0519)
  arc A124 (-106.7156, -25.841) -> (-106.4227, -25.1339) centre (-107.4227, -25.1339) ccw
  arc A125 (-111.4227, -25.1339) -> (-111.1298, -25.841) centre (-110.4227, -25.1339) ccw
  line L310 (-106.7156, -25.841) -> (-108.6227, -27.7481)
  line L311 (-111.1298, -25.841) -> (-109.2227, -27.7481)
  line L312 (-108.9227, -27.7481) -> (-108.6227, -27.7481)
  line L313 (-108.9227, -27.7481) -> (-109.2227, -27.7481)
  line L314 (-111.4227, -25.1339) -> (-111.4227, -8.3624)
  line L315 (-106.4227, -8.3624) -> (-106.4227, -25.1339)
  arc A126 (-111.1298, -7.6553) -> (-111.4227, -8.3624) centre (-110.4227, -8.3624) ccw
  line L316 (-111.1298, -7.6553) -> (-109.2227, -5.7481)
  line L317 (-108.9227, -5.7481) -> (-109.2227, -5.7481)
  line L318 (-108.9227, -5.7481) -> (-108.6227, -5.7481)
  arc A127 (-106.4227, -8.3624) -> (-106.7156, -7.6553) centre (-107.4227, -8.3624) ccw
  line L319 (-106.7156, -7.6553) -> (-108.6227, -5.7481)
  arc A128 (-81.9156, -1.041) -> (-81.6227, -0.3339) centre (-82.6227, -0.3339) ccw
  arc A129 (-86.6227, -0.3339) -> (-86.3298, -1.041) centre (-85.6227, -0.3339) ccw
  line L320 (-81.9156, -1.041) -> (-83.8227, -2.9481)
  line L321 (-86.3298, -1.041) -> (-84.4227, -2.9481)
  line L322 (-84.1227, -2.9481) -> (-83.8227, -2.9481)
  line L323 (-84.1227, -2.9481) -> (-84.4227, -2.9481)
  line L324 (-86.6227, -0.3339) -> (-86.6227, 16.4376)
  line L325 (-81.6227, 16.4376) -> (-81.6227, -0.3339)
  arc A130 (-86.3298, 17.1447) -> (-86.6227, 16.4376) centre (-85.6227, 16.4376) ccw
  line L326 (-86.3298, 17.1447) -> (-84.4227, 19.0519)
  line L327 (-84.1227, 19.0519) -> (-84.4227, 19.0519)
  line L328 (-84.1227, 19.0519) -> (-83.8227, 19.0519)
  arc A131 (-81.6227, 16.4376) -> (-81.9156, 17.1447) centre (-82.6227, 16.4376) ccw
  line L329 (-81.9156, 17.1447) -> (-83.8227, 19.0519)
  arc A132 (-81.9156, -25.841) -> (-81.6227, -25.1339) centre (-82.6227, -25.1339) ccw
  arc A133 (-86.6227, -25.1339) -> (-86.3298, -25.841) centre (-85.6227, -25.1339) ccw
  line L330 (-81.9156, -25.841) -> (-83.8227, -27.7481)
  line L331 (-86.3298, -25.841) -> (-84.4227, -27.7481)
  line L332 (-84.1227, -27.7481) -> (-83.8227, -27.7481)
  line L333 (-84.1227, -27.7481) -> (-84.4227, -27.7481)
  line L334 (-86.6227, -25.1339) -> (-86.6227, -8.3624)
  line L335 (-81.6227, -8.3624) -> (-81.6227, -25.1339)
  arc A134 (-86.3298, -7.6553) -> (-86.6227, -8.3624) centre (-85.6227, -8.3624) ccw
  line L336 (-86.3298, -7.6553) -> (-84.4227, -5.7481)
  line L337 (-84.1227, -5.7481) -> (-84.4227, -5.7481)
  line L338 (-84.1227, -5.7481) -> (-83.8227, -5.7481)
  arc A135 (-81.6227, -8.3624) -> (-81.9156, -7.6553) centre (-82.6227, -8.3624) ccw
  line L339 (-81.9156, -7.6553) -> (-83.8227, -5.7481)
  arc A136 (-105.6156, -31.3553) -> (-104.9084, -31.6481) centre (-104.9084, -30.6481) ccw
  arc A137 (-104.9084, -26.6481) -> (-105.6156, -26.941) centre (-104.9084, -27.6481) ccw
  line L340 (-105.6156, -31.3553) -> (-107.5227, -29.4481)
  line L341 (-105.6156, -26.941) -> (-107.5227, -28.8481)
  line L342 (-107.5227, -29.1481) -> (-107.5227, -29.4481)
  line L343 (-107.5227, -29.1481) -> (-107.5227, -28.8481)
  line L344 (-104.9084, -26.6481) -> (-88.1369, -26.6481)
  line L345 (-88.1369, -31.6481) -> (-104.9084, -31.6481)
  arc A138 (-87.4298, -26.941) -> (-88.1369, -26.6481) centre (-88.1369, -27.6481) ccw
  line L346 (-87.4298, -26.941) -> (-85.5227, -28.8481)
  line L347 (-85.5227, -29.1481) -> (-85.5227, -28.8481)
  line L348 (-85.5227, -29.1481) -> (-85.5227, -29.4481)
  arc A139 (-88.1369, -31.6481) -> (-87.4298, -31.3553) centre (-88.1369, -30.6481) ccw
  line L349 (-87.4298, -31.3553) -> (-85.5227, -29.4481)
  arc A140 (99.8844, 18.2447) -> (100.5916, 17.9519) centre (100.5916, 18.9519) ccw
  arc A141 (100.5916, 22.9519) -> (99.8844, 22.659) centre (100.5916, 21.9519) ccw
  line L350 (99.8844, 18.2447) -> (97.9773, 20.1519)
  line L351 (99.8844, 22.659) -> (97.9773, 20.7519)
  line L352 (97.9773, 20.4519) -> (97.9773, 20.1519)
  line L353 (97.9773, 20.4519) -> (97.9773, 20.7519)
  line L354 (100.5916, 22.9519) -> (117.3631, 22.9519)
  line L355 (117.3631, 17.9519) -> (100.5916, 17.9519)
  arc A142 (118.0702, 22.659) -> (117.3631, 22.9519) centre (117.3631, 21.9519) ccw
  line L356 (118.0702, 22.659) -> (119.9773, 20.7519)
  line L357 (119.9773, 20.4519) -> (119.9773, 20.7519)
  line L358 (119.9773, 20.4519) -> (119.9773, 20.1519)
  arc A143 (117.3631, 17.9519) -> (118.0702, 18.2447) centre (117.3631, 18.9519) ccw
  line L359 (118.0702, 18.2447) -> (119.9773, 20.1519)
  arc A144 (99.8844, -6.5553) -> (100.5916, -6.8481) centre (100.5916, -5.8481) ccw
  arc A145 (100.5916, -1.8481) -> (99.8844, -2.141) centre (100.5916, -2.8481) ccw
  line L360 (99.8844, -6.5553) -> (97.9773, -4.6481)
  line L361 (99.8844, -2.141) -> (97.9773, -4.0481)
  line L362 (97.9773, -4.3481) -> (97.9773, -4.6481)
  line L363 (97.9773, -4.3481) -> (97.9773, -4.0481)
  line L364 (100.5916, -1.8481) -> (117.3631, -1.8481)
  line L365 (117.3631, -6.8481) -> (100.5916, -6.8481)
  arc A146 (118.0702, -2.141) -> (117.3631, -1.8481) centre (117.3631, -2.8481) ccw
  line L366 (118.0702, -2.141) -> (119.9773, -4.0481)
  line L367 (119.9773, -4.3481) -> (119.9773, -4.0481)
  line L368 (119.9773, -4.3481) -> (119.9773, -4.6481)
  arc A147 (117.3631, -6.8481) -> (118.0702, -6.5553) centre (117.3631, -5.8481) ccw
  line L369 (118.0702, -6.5553) -> (119.9773, -4.6481)
  arc A148 (98.7844, -1.041) -> (99.0773, -0.3339) centre (98.0773, -0.3339) ccw
  arc A149 (94.0773, -0.3339) -> (94.3702, -1.041) centre (95.0773, -0.3339) ccw
  line L370 (98.7844, -1.041) -> (96.8773, -2.9481)
  line L371 (94.3702, -1.041) -> (96.2773, -2.9481)
  line L372 (96.5773, -2.9481) -> (96.8773, -2.9481)
  line L373 (96.5773, -2.9481) -> (96.2773, -2.9481)
  line L374 (94.0773, -0.3339) -> (94.0773, 16.4376)
  line L375 (99.0773, 16.4376) -> (99.0773, -0.3339)
  arc A150 (94.3702, 17.1447) -> (94.0773, 16.4376) centre (95.0773, 16.4376) ccw
  line L376 (94.3702, 17.1447) -> (96.2773, 19.0519)
  line L377 (96.5773, 19.0519) -> (96.2773, 19.0519)
  line L378 (96.5773, 19.0519) -> (96.8773, 19.0519)
  arc A151 (99.0773, 16.4376) -> (98.7844, 17.1447) centre (98.0773, 16.4376) ccw
  line L379 (98.7844, 17.1447) -> (96.8773, 19.0519)
  arc A152 (98.7844, -25.841) -> (99.0773, -25.1339) centre (98.0773, -25.1339) ccw
  arc A153 (94.0773, -25.1339) -> (94.3702, -25.841) centre (95.0773, -25.1339) ccw
  line L380 (98.7844, -25.841) -> (96.8773, -27.7481)